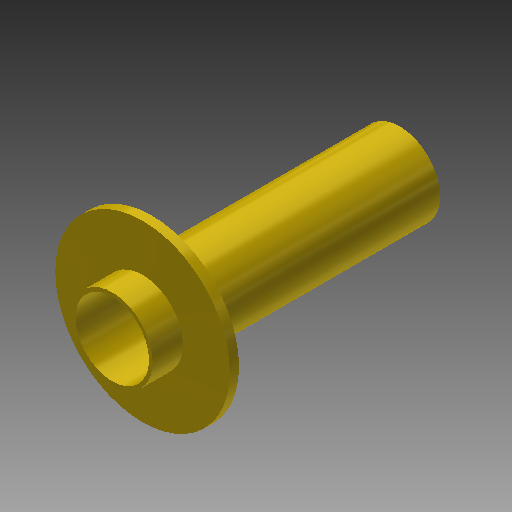
# Autodesk Inventor part: ALPHA_001161_ExitTube
Saved by Autodesk Inventor 2017 (Build 210142000, 142)
## iProperties
Created: 2015-11-18
Part Number: ALPHA_001161_ExitTube
Material: Generic
Document SubType Name: Modeling
Designer: massen
Density: 1 g/cm^3
Appearance: Glossy - Gold
Author: massen
Autodesk Inventor part; units mm, degrees
ref_plane "YZ Plane" through (0, 0, 0) normal (1, 0, 0) x (0, 1, 0)
ref_plane "XZ Plane" through (0, 0, 0) normal (0, 1, 0) x (-1, 0, 0)
ref_plane "XY Plane" through (0, 0, 0) normal (0, 0, 1) x (1, 0, 0)
sketch "Sketch1" plane through (0, 0, 0) normal (0, 0, 1) x (1, 0, 0)
  circle A0 centre (0, 0) radius 20
  circle A1 centre (0, 0) radius 22
  circle A2 centre (0, 0) radius 47.5
  circle A3 centre (0, 0) radius 37.5 construction
  dimension "d0" = 40
  dimension "d1" = 44
  dimension "d2" = 95
  dimension "d3" = 75
  constraints: 4 centre point, 4 coincident
  measures "d0" diameter of A0
  measures "d1" diameter of A1
  measures "d2" diameter of A2
  measures "d3" diameter of A3
extrude "Extrusion1" add sketch "Sketch1" along normal blind 16.5 and the other way blind 140 contours A1
extrude "Extrusion2" add sketch "Sketch1" against normal blind 5 contours A2
body "Solid1"
